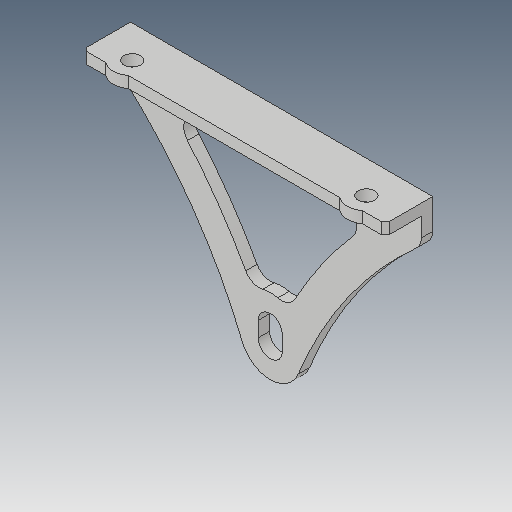
# Autodesk Inventor part: NUC_tab
Saved by Autodesk Inventor 2019.4 (Build 234330000, 330)
## iProperties
Created: 2019-01-20
Part Number: NUC_tab
Material: 一般
Document SubType Name: Modeling
Designer: y6tada
Density: 1 g/cm^3
Appearance: 既定
Mass: 0.943627 g
Surface Area: 15.8128 cm^2
Volume: 0.943627 cm^3
Author: y6tada
Autodesk Inventor part; units mm, degrees
ref_plane "YZ Plane" through (0, 0, 0) normal (1, 0, 0) x (0, 1, 0)
ref_plane "XZ Plane" through (0, 0, 0) normal (0, 1, 0) x (-1, 0, 0)
ref_plane "XY Plane" through (0, 0, 0) normal (0, 0, 1) x (1, 0, 0)
sketch "スケッチ1" plane through (0, 0, 0) normal (0, 0, 1) x (1, 0, 0)
  line L0 (-59, -17.25) -> (53, -17.25) construction
  line L1 (1.6, -41.5) -> (-1.6, -41.5) construction
  line L2 (-1.6, -41.5) -> (-1.6, -43.5)
  line L3 (-1.6, -43.5) -> (1.6, -43.5) construction
  line L4 (1.6, -43.5) -> (1.6, -41.5)
  arc A0 (1.6, -41.5) -> (-1.6, -41.5) centre (0, -41.5) ccw
  arc A1 (-1.6, -43.5) -> (1.6, -43.5) centre (0, -43.5) ccw
  circle A2 centre (0, -42.5) radius 1.5 construction
  line L5 (0, -41.5) -> (0, -42.5) construction
  line L6 (0, -42.5) -> (0, -43.5) construction
  line L7 (0, -41.5) -> (0, -17.25) construction
  line L8 (0, -17.25) -> (-20, -17.25)
  line L9 (-20, -17.25) -> (-20, -21.25)
  line L10 (0, -17.25) -> (20, -17.25)
  line L11 (20, -17.25) -> (20, -21.25)
  arc A3 (-3.7095, -44.9966) -> (3.7095, -44.9966) centre (0, -43.5) ccw
  arc A4 (-3.7095, -44.9966) -> (-19.3339, -22.7402) centre (-59.3515, -67.4458) ccw
  arc A5 (19.3339, -22.7402) -> (3.7095, -44.9966) centre (59.3515, -67.4458) ccw
  arc A6 (-20, -21.25) -> (-19.3339, -22.7402) centre (-18, -21.25) ccw
  arc A7 (19.3339, -22.7402) -> (20, -21.25) centre (18, -21.25) ccw
  arc A8 (-3.2471, -36.6513) -> (-10.9625, -25.559) centre (-59.3515, -67.4458) ccw
  arc A9 (10.9625, -25.559) -> (3.2471, -36.6513) centre (59.3515, -67.4458) ccw
  arc A10 (0.9959, -37.626) -> (-0.9959, -37.626) centre (0, -41.5) ccw
  line L12 (-9.4504, -22.25) -> (9.4504, -22.25)
  arc A11 (-9.4504, -22.25) -> (-10.9625, -25.559) centre (-9.4504, -24.25) ccw
  arc A12 (10.9625, -25.559) -> (9.4504, -22.25) centre (9.4504, -24.25) ccw
  arc A13 (0.9959, -37.626) -> (3.2471, -36.6513) centre (1.4939, -35.6889) ccw
  arc A14 (-3.2471, -36.6513) -> (-0.9959, -37.626) centre (-1.4939, -35.6889) ccw
  point P0 (0, 0)
  point P1 (-20, -22.1528)
  point P2 (20, -22.1528)
  dimension "d0" = 2
  dimension "d1" = 1.6
  dimension "d3" = 4
  dimension "d4" = 2
  dimension "d5" = 4
  dimension "d6" = 60
  dimension "d7" = 20
  dimension "d8" = 4
  dimension "d9" = 4
  dimension "d10" = 2.4
  dimension "d11" = 5
  dimension "d12" = 2
  constraints: 30 point on circle, 24 end point, 14 centre point, 14 tangent, 5 equal radius, 5 point on line, 5 vertical, 3 equal length, 3 parallel, 2 midpoint, 1 concentric, 1 horizontal, 1 perpendicular
  measures "d0" distance of L1.end L2.end
  measures "d1" radius of A0
  measures "d3" radius of A3
  measures "d4" radius of A6
  measures "d5" distance of L10.end L11.end
  measures "d6" radius of A5
  measures "d7" distance of L7.end L8.end
  measures "d8" radial gap between concentric circles of A4 A8
  measures "d9" radial gap between concentric circles of A5 A9
  measures "d10" radial gap between concentric circles of A0 A10
  measures "d11" distance between parallel lines of L0 L12
  measures "d12" radius of A11
extrude "押し出し1" add sketch "スケッチ1" against normal blind 1.5
sketch "スケッチ2" plane through (-20, -17.25, 0) normal (0, 1, 0) x (1, 0, 0)
  line L0 (40, 0) -> (0, 0) construction
  line L1 (40, 0) -> (0, 0)
  line L2 (0, 0) -> (0, -4.2744)
  line L3 (0.5, -4.7744) -> (3, -4.7744)
  line L4 (40, -4.2744) -> (40, 0)
  line L5 (0, 0) -> (0, 1.5) construction
  line L6 (69.5882, -4.7744) -> (-3.4118, -4.7744) construction
  line L7 (20, 0) -> (20, -8.2375) construction
  circle A0 centre (35.5, -2.7744) radius 1.1
  line L8 (40, -4.2744) -> (39.5, -4.7744)
  line L9 (0.5, -4.7744) -> (0, -4.2744)
  arc A1 (34, -4.7744) -> (37, -4.7744) centre (35.5, -2.7744) ccw
  line L10 (37, -4.7744) -> (39.5, -4.7744)
  line L11 (34, -4.7744) -> (37, -4.7744) construction
  circle A2 centre (4.5, -2.7744) radius 1.1
  arc A3 (3, -4.7744) -> (6, -4.7744) centre (4.5, -2.7744) ccw
  line L12 (6, -4.7744) -> (34, -4.7744)
  line L13 (3, -4.7744) -> (6, -4.7744) construction
  point P0 (40, -4.7744)
  point P1 (0, -4.7744)
  dimension "d18" = 2.2
  dimension "d19" = 0.5
  dimension "d20" = 0.5
  dimension "d21" = 0.5
  dimension "d22" = 0.5
  dimension "d23" = 2.5
  dimension "d24" = 4.5
  dimension "d25" = 2
  constraints: 22 end point, 6 collinear, 6 parallel, 6 point on line, 4 centre point, 4 point on circle, 4 symmetric about line, 1 concentric, 1 horizontal, 1 perpendicular, 1 vertical, 2 other
  measures "d18" diameter of A0
  measures "d19" distance of L4.start point (40, -4.774)
  measures "d20" distance of L8.end point (40, -4.774)
  measures "d21" distance of L3.start point (0, -4.774)
  measures "d22" distance of L2.end point (0, -4.774)
  measures "d23" radius of A1
  measures "d24" distance from line of L4 A0.centre
  measures "d25" distance from line of L3 A0.centre
extrude "押し出し2" add sketch "スケッチ2" against normal blind 1.5
equation "\"d20\" = d19"
equation "\"d21\" = d19"
equation "\"d22\" = d21"
